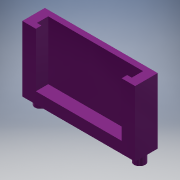
# Autodesk Inventor part: CameraMount
Saved by Autodesk Inventor 2018 (Build 220112000, 112)
## iProperties
Created: 2018-01-13
Part Number: CameraMount
Material: ABS Plastic
Document SubType Name: Modeling
Designer: Kyle-HP
Density: 1.06 g/cm^3
Appearance: Smooth - Purple
Author: Kyle-HP
Autodesk Inventor part; units mm, degrees
ref_plane "YZ Plane" through (0, 0, 0) normal (1, 0, 0) x (0, 1, 0)
ref_plane "XZ Plane" through (0, 0, 0) normal (0, 1, 0) x (-1, 0, 0)
ref_plane "XY Plane" through (0, 0, 0) normal (0, 0, 1) x (1, 0, 0)
sketch "Sketch1" plane through (0, 0, 0) normal (0, 0, 1) x (1, 0, 0)
  line L0 (0, 0) -> (31.75, 0)
  line L1 (31.75, 0) -> (31.75, -18.415)
  line L2 (31.75, -18.415) -> (0, -18.415)
  line L3 (0, -18.415) -> (0, 0)
  dimension "d0" = 31.75
  dimension "d1" = 18.415
  constraints: 8 end point, 2 parallel, 1 horizontal, 1 perpendicular
  measures "d0" distance of L0.start L0.end
  measures "d1" distance of L0.end L1.end
extrude "Extrusion1" add sketch "Sketch1" along normal blind 6.35
sketch "Sketch2" plane through (0, 0, 0) normal (0, 1, 0) x (1, 0, 0)
  line L0 (2.54, -1.5875) -> (29.21, -1.5875)
  line L1 (29.21, -1.5875) -> (29.21, -4.7625)
  line L2 (29.21, -4.7625) -> (2.54, -4.7625)
  line L3 (2.54, -4.7625) -> (2.54, -1.5875)
  line L4 (0, 0) -> (0, -6.35) projected
  line L5 (31.75, -6.35) -> (0, -6.35) projected
  dimension "d4" = 26.67
  dimension "d5" = 2.54
  dimension "d6" = 3.175
  dimension "d7" = 1.5875
  constraints: 8 end point, 2 parallel, 1 horizontal, 1 perpendicular
  measures "d4" distance of L1.end L2.end
  measures "d5" distance between parallel lines of L4 L3
  measures "d6" distance of L2.end L0.start
  measures "d7" distance between parallel lines of L5 L2
extrude "Extrusion2" cut sketch "Sketch2" against normal blind 16.51
sketch "Sketch3" plane through (29.21, 0, 4.7625) normal (0, 0, -1) x (-1, 0, 0)
  line L0 (1.27, 0) -> (25.4, 0)
  line L1 (25.4, 0) -> (25.4, -15.24)
  line L2 (25.4, -15.24) -> (1.27, -15.24)
  line L3 (1.27, -15.24) -> (1.27, 0)
  line L4 (26.67, -16.51) -> (0, -16.51) projected
  line L5 (26.67, 0) -> (26.67, -16.51) projected
  line L6 (0, 0) -> (0, -16.51) projected
  line L7 (0, 0) -> (26.67, 0) projected
  point P0 (29.21, 0)
  dimension "d10" = 1.27
  dimension "d11" = 1.27
  dimension "d12" = 1.27
  dimension "d13" = 0
  constraints: 8 end point, 2 parallel, 1 horizontal, 1 perpendicular
  measures "d10" distance between parallel lines of L2 L4
  measures "d11" distance between parallel lines of L1 L5
  measures "d12" distance between parallel lines of L3 L6
  measures "d13" distance between parallel lines of L7 L0
extrude "Extrusion3" cut sketch "Sketch3" against normal blind 16.51 contours L0 L1 L2 L3
sketch "Sketch4" plane through (0, -18.415, 0) normal (0, -1, 0) x (1, 0, 0)
  circle A0 centre (1.905, 3.175) radius 1.5621
  circle A1 centre (29.845, 3.175) radius 1.5621
  line L0 (0, 6.35) -> (31.75, 6.35) projected
  line L1 (0, 0) -> (0, 6.35) projected
  dimension "d16" = 3.1242
  dimension "d17" = 3.1242
  dimension "d18" = 3.175
  dimension "d19" = 3.175
  dimension "d20" = 27.94
  dimension "d21" = 1.905
  constraints: 2 centre point
  measures "d16" diameter of A1
  measures "d17" diameter of A0
  measures "d18" distance from line of L0 A0.centre
  measures "d19" distance from line of L0 A1.centre
  measures "d20" distance of A0.centre A1.centre
  measures "d21" distance from line of L1 A0.centre
extrude "Extrusion4" add sketch "Sketch4" along normal blind 2.54
body "Solid1"
